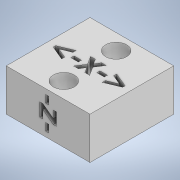
# Autodesk Inventor part: squareCalibrationBlock-25mm
Saved by Autodesk Inventor 2020.3 (Build 243373000, 373)
## iProperties
Created: 2020-06-02
Part Number: squareCalibrationBlock-25mm
Material: Generic
Document SubType Name: Modeling
Designer: robst
Density: 1 g/cm^3
Appearance: Default
Author: robst
Autodesk Inventor part; units mm, degrees
ref_plane "YZ Plane" through (0, 0, 0) normal (1, 0, 0) x (0, 1, 0)
ref_plane "XZ Plane" through (0, 0, 0) normal (0, 1, 0) x (-1, 0, 0)
ref_plane "XY Plane" through (0, 0, 0) normal (0, 0, 1) x (1, 0, 0)
sketch "Sketch1" plane through (0, 0, 0) normal (0, 1, 0) x (-1, 0, 0)
  line L0 (12.7, 12.7) -> (-12.7, 12.7)
  line L1 (-12.7, 12.7) -> (-12.7, -12.7)
  line L2 (-12.7, -12.7) -> (12.7, -12.7)
  line L3 (12.7, -12.7) -> (12.7, 12.7)
  line L4 (12.7, 12.7) -> (-12.7, -12.7) construction
  line L5 (-12.7, 12.7) -> (12.7, -12.7) construction
  point P0 (0, 0)
  dimension "d0" = 25.4
  dimension "d1" = 25.4
  constraints: 12 end point, 2 midpoint, 2 parallel, 1 horizontal, 1 perpendicular
  measures "d0" distance of L0.start L0.end
  measures "d1" distance of L1.end L0.end
extrude "Extrusion1" add sketch "Sketch1" along normal blind 12.7
sketch "Sketch2" plane through (0, 12.7, 0) normal (0, 1, 0) x (1, 0, 0)
  line L0 (-12.7, 12.7) -> (-12.7, -12.7) construction
  line L1 (-12.7, 0) -> (12.7, 0) construction
  line L2 (12.7, -12.7) -> (12.7, 12.7) construction
  line L3 (-6.1256, -2.4906) -> (-10.5058, -0.671)
  line L4 (-10.5058, -0.671) -> (-10.5058, 0.0782)
  line L5 (-10.5058, 0.0782) -> (-6.1256, 1.8978)
  line L6 (-6.1256, 1.8978) -> (-6.1256, 0.9551)
  line L7 (-6.1256, 0.9551) -> (-9.1885, -0.3005)
  line L8 (-9.1885, -0.3005) -> (-6.1256, -1.5479)
  line L9 (-6.1256, -1.5479) -> (-6.1256, -2.4906)
  line L10 (-2.7705, -0.7698) -> (-5.0306, -0.7698)
  line L11 (-5.0306, -0.7698) -> (-5.0306, 0.177)
  line L12 (-5.0306, 0.177) -> (-2.7705, 0.177)
  line L13 (-2.7705, 0.177) -> (-2.7705, -0.7698)
  line L14 (2.433, -2.54) -> (0.9592, -2.54)
  line L15 (0.9592, -2.54) -> (-0.0206, -0.9221)
  line L16 (-0.0206, -0.9221) -> (-1.0209, -2.54)
  line L17 (-1.0209, -2.54) -> (-2.433, -2.54)
  line L18 (-2.433, -2.54) -> (-0.7822, 0.0165)
  line L19 (-0.7822, 0.0165) -> (-2.3671, 2.54)
  line L20 (-2.3671, 2.54) -> (-0.8933, 2.54)
  line L21 (-0.8933, 2.54) -> (0.0247, 1.0045)
  line L22 (0.0247, 1.0045) -> (0.9674, 2.54)
  line L23 (0.9674, 2.54) -> (2.3794, 2.54)
  line L24 (2.3794, 2.54) -> (0.7863, 0.07)
  line L25 (0.7863, 0.07) -> (2.433, -2.54)
  line L26 (5.1088, -0.7698) -> (2.8488, -0.7698)
  line L27 (2.8488, -0.7698) -> (2.8488, 0.177)
  line L28 (2.8488, 0.177) -> (5.1088, 0.177)
  line L29 (5.1088, 0.177) -> (5.1088, -0.7698)
  line L30 (10.5881, -0.671) -> (6.208, -2.4906)
  line L31 (6.208, -2.4906) -> (6.208, -1.5479)
  line L32 (6.208, -1.5479) -> (9.2667, -0.2964)
  line L33 (9.2667, -0.2964) -> (6.208, 0.9551)
  line L34 (6.208, 0.9551) -> (6.208, 1.8978)
  line L35 (6.208, 1.8978) -> (10.5881, 0.0782)
  line L36 (10.5881, 0.0782) -> (10.5881, -0.671)
  point P0 (0, 0)
  constraints: 2 end point, 2 midpoint, 1 horizontal
extrude "Extrusion2" cut sketch "Sketch2" against normal blind 5.08
sketch "Sketch3" plane through (-12.7, 0, 12.7) normal (0, 0, 1) x (1, 0, 0)
  line L0 (12.6794, 12.7) -> (11.6791, 12.7) construction
  line L1 (12.7, 0) -> (12.6794, 12.7) construction
  line L2 (11.9158, 8.9011) -> (11.9121, 11.1612)
  line L3 (11.9121, 11.1612) -> (12.8589, 11.1627)
  line L4 (12.8589, 11.1627) -> (12.8626, 8.9026)
  line L5 (12.8626, 8.9026) -> (11.9158, 8.9011)
  line L6 (10.153, 4.3081) -> (10.1465, 8.3342)
  line L7 (10.1465, 8.3342) -> (11.0974, 8.3358)
  line L8 (11.0974, 8.3358) -> (14.2629, 5.9985)
  line L9 (14.2629, 5.9985) -> (14.2593, 8.2174)
  line L10 (14.2593, 8.2174) -> (15.2267, 8.219)
  line L11 (15.2267, 8.219) -> (15.2328, 4.4522)
  line L12 (15.2328, 4.4522) -> (14.2654, 4.4506)
  line L13 (14.2654, 4.4506) -> (11.1164, 6.7797)
  line L14 (11.1164, 6.7797) -> (11.1204, 4.3097)
  line L15 (11.1204, 4.3097) -> (10.153, 4.3081)
  line L16 (11.9277, 1.5405) -> (11.924, 3.8005)
  line L17 (11.924, 3.8005) -> (12.8709, 3.8021)
  line L18 (12.8709, 3.8021) -> (12.8745, 1.542)
  line L19 (12.8745, 1.542) -> (11.9277, 1.5405)
  constraints: 2 end point, 1 other
extrude "Extrusion3" cut sketch "Sketch3" against normal blind 5.08
sketch "Sketch11" plane through (0, 12.7, 0) normal (0, 1, 0) x (1, 0, 0)
  circle A0 centre (0, 7.9375) radius 3.175
  circle A1 centre (0, -7.9375) radius 3.175
  line L0 (12.7, 12.7) -> (-12.7, 12.7) projected
  line L1 (-12.7, -12.7) -> (12.7, -12.7) projected
  point P0 (0, 0)
  dimension "d81" = 6.35
  dimension "d82" = 4.7625
  dimension "d83" = 4.7625
  constraints: 2 centre point, 1 equal radius
  measures "d81" diameter of A0
  measures "d82" distance from line of A0.centre L0
  measures "d83" distance from line of A1.centre L1
extrude "Extrusion4" cut sketch "Sketch11" against normal blind 25.4
equation "\"d46\" = 0.125 * Sketch7_Pitch"
equation "\"Sketch7_Pitch\" = 1.27"
equation "\"d48\" = 60deg"
equation "\"d67\" = 0.125 * Sketch9_Pitch"
equation "\"Sketch9_Pitch\" = 1.27"
equation "\"d69\" = 60deg"
equation "\"d99\" = 0.125 * Sketch12_Pitch"
equation "\"Sketch12_Pitch\" = 1.27"
equation "\"d101\" = 60deg"
equation "\"d120\" = 0.125 * Sketch14_Pitch"
equation "\"Sketch14_Pitch\" = 1.27"
equation "\"d122\" = 60deg"
equation "\"d143\" = 55deg"
equation "\"Sketch16_Pitch\" = 1.27"
equation "\"d161\" = 55deg"
equation "\"Sketch18_Pitch\" = 1.27"
body "Solid1"
